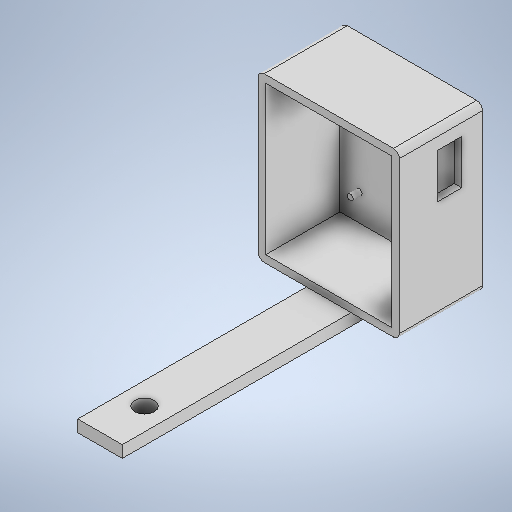
# Autodesk Inventor part: a4988_box
Saved by Autodesk Inventor 2025 (Build 290162000, 162)
## iProperties
Created: 2025-03-03
Part Number: a4988_box
Material: Všeobecné
Document SubType Name: Modeling
Designer: lukas
Density: 1 g/cm^3
Appearance: Výchozí
Author: lukas
## iProperties of the stored document a4988_box_3D tisk.ipt
Created: 2025-03-03
Part Number: a4988_box_3D tisk
Material: Všeobecné
Document SubType Name: Modeling
Designer: lukas
Density: 1 g/cm^3
Appearance: Výchozí
Author: lukas
Autodesk Inventor part; units mm, degrees
ref_plane "YZ Plane" through (0, 0, 0) normal (1, 0, 0) x (0, 1, 0)
ref_plane "XZ Plane" through (0, 0, 0) normal (0, 1, 0) x (-1, 0, 0)
ref_plane "XY Plane" through (0, 0, 0) normal (0, 0, 1) x (1, 0, 0)
sketch "Náčrt1" plane through (0, 0, 0) normal (0, 0, 1) x (1, 0, 0)
  line L0 (-21.25, 25) -> (21.25, 25)
  line L1 (21.25, 25) -> (21.25, -25)
  line L2 (21.25, -25) -> (-21.25, -25)
  line L3 (-21.25, -25) -> (-21.25, 25)
  line L4 (0, 35) -> (0, -35) projected
  line L5 (-29.75, 0) -> (29.75, 0) projected
  point P0 (0, 0)
  dimension "d0" = 50
  dimension "d1" = 42.5
  constraints: 8 end point, 2 parallel, 1 horizontal, 1 perpendicular, 2 other
  measures "d0" distance between parallel lines of L2 L0
  measures "d1" distance between parallel lines of L3 L1
extrude "Vysunutí1" add sketch "Náčrt1" along normal blind 3
sketch "Náčrt2" plane through (0, 0, 3) normal (0, 0, 1) x (1, 0, 0)
  line L0 (0, 35) -> (0, -35) projected
  line L1 (-29.75, 0) -> (29.75, 0) projected
  line L2 (21.25, -25) -> (21.25, 25) projected
  line L3 (21.25, 25) -> (-21.25, 25) projected
  line L4 (-21.25, 25) -> (-21.25, -25) projected
  line L5 (-21.25, -25) -> (21.25, -25) projected
  line L6 (-17.5, 21.5) -> (17.5, 21.5) construction
  line L7 (17.5, 21.5) -> (17.5, -21.5) construction
  line L8 (17.5, -21.5) -> (-17.5, -21.5) construction
  line L9 (-17.5, -21.5) -> (-17.5, 21.5) construction
  circle A0 centre (-14.75, 16) radius 1
  circle A1 centre (-14.75, -16) radius 1
  point P0 (0, 0)
  dimension "d4" = 35
  dimension "d5" = 43
  dimension "d6" = 2
  dimension "d9" = 16
  dimension "d10" = 36
  constraints: 8 end point, 2 centre point, 2 parallel, 1 horizontal, 1 perpendicular, 1 symmetric about line, 3 other
  measures "d4" distance of L6.start L6.end
  measures "d5" distance of L6.end L7.end
  measures "d6" diameter of A0
  measures "d9" distance from line of L1 A0.centre
  measures "d10" distance from line of L2 A0.centre
extrude "Vysunutí2" add sketch "Náčrt2" along normal blind 3 contours A0 | A1
sketch "Náčrt3" plane through (0, 0, 3) normal (0, 0, 1) x (1, 0, 0)
  circle A0 centre (-14.75, -16) radius 1 projected
  circle A1 centre (-14.75, 16) radius 1 projected
  line L0 (21.25, -25) -> (21.25, 25) projected
  line L1 (21.25, 25) -> (-21.25, 25) projected
  line L2 (-21.25, 25) -> (-21.25, -25) projected
  line L3 (-21.25, -25) -> (21.25, -25) projected
  line L4 (0, 35) -> (0, -35) projected
  line L5 (-29.75, 0) -> (29.75, 0) projected
  line L6 (-23.75, 27.5) -> (23.75, 27.5)
  line L7 (23.75, 27.5) -> (23.75, -27.5)
  line L8 (23.75, -27.5) -> (-23.75, -27.5)
  line L9 (-23.75, -27.5) -> (-23.75, 27.5)
  line L10 (-21.25, 25) -> (21.25, 25)
  line L11 (21.25, 25) -> (21.25, -25)
  line L12 (21.25, -25) -> (-21.25, -25)
  line L13 (-21.25, -25) -> (-21.25, 25)
  point P0 (0, 0)
  dimension "d13" = 2.5
  constraints: 16 end point, 2 parallel, 1 horizontal, 1 perpendicular, 3 other
  measures "d13" distance between parallel lines of L1 L6
extrude "Vysunutí3" add sketch "Náčrt3" along normal blind 25 and the other way blind 3 contours L0 L5 L7 L8 L4 L3 | L0 L1 L4 L6 L7 L5 | L4 L8 L9 L5 L2 L3 | L1 L2 L5 L9 L6 L4
sketch "Náčrt4" plane through (23.75, -27.5, 28) normal (1, 0, 0) x (0, 0, -1)
  line L0 (13, 34) -> (21, 34)
  line L1 (21, 34) -> (21, 49)
  line L2 (21, 49) -> (13, 49)
  line L3 (13, 49) -> (13, 34)
  line L4 (0, 55) -> (28, 55) projected
  line L5 (0, 0) -> (0, 55) projected
  line L6 (28, 0) -> (0, 0) projected
  line L7 (28, 55) -> (28, 0) projected
  line L8 (-6.6, 27.5) -> (39.6, 27.5) projected
  line L9 (28, -11) -> (28, 66) projected
  line L10 (25, 2.5) -> (25, 52.5) projected
  line L11 (0, 52.5) -> (25, 52.5) projected
  point P0 (28, 27.5)
  dimension "d18" = 15
  dimension "d19" = 8
  dimension "d20" = 7
  dimension "d21" = 6
  constraints: 8 end point, 2 parallel, 1 horizontal, 1 perpendicular
  measures "d18" distance of L2.end L0.start
  measures "d19" distance of L0.start L0.end
  measures "d20" distance between parallel lines of L7 L1
  measures "d21" distance between parallel lines of L4 L2
extrude "Vysunutí4" cut sketch "Náčrt4" against normal up to surface (2.5 mm away) contours L3 L2 L1 L0
sketch "Náčrt5" plane through (-23.75, -27.5, 28) normal (0, -1, 0) x (1, 0, 0)
  line L0 (47.5, -28) -> (47.5, 0) projected
  line L1 (0, 0) -> (47.5, 0) projected
  line L2 (0, -28) -> (0, 0) projected
  line L3 (47.5, -28) -> (0, -28) projected
  line L4 (23.75, 99) -> (23.75, -55) projected
  line L5 (-9.5, -28) -> (57, -28) projected
  line L6 (31.25, -28) -> (16.25, -28)
  line L7 (16.25, -28) -> (16.25, 77)
  line L8 (16.25, 77) -> (31.25, 77)
  line L9 (31.25, 77) -> (31.25, -28)
  point P0 (23.75, -28)
  point P1 (31.25, -28)
  dimension "d24" = 15
  dimension "d25" = 77
  constraints: 8 end point, 2 parallel, 1 horizontal, 1 perpendicular, 1 point on line, 1 other
  measures "d24" distance between parallel lines of L9 L7
  measures "d25" distance between parallel lines of L1 L8
extrude "Vysunutí5" add sketch "Náčrt5" along normal blind 5 contours L3 L4 L1 L9 | L1 L4 L8 L9 | L3 L7 L1 L4 | L1 L7 L8 L4
sketch "Náčrt6" plane through (-23.75, -32.5, 28) normal (0, -1, 0) x (1, 0, 0)
  line L0 (16.25, 77) -> (16.25, -28) projected
  line L1 (16.25, -28) -> (31.25, -28) projected
  line L2 (31.25, -28) -> (31.25, 77) projected
  line L3 (31.25, 77) -> (16.25, 77) projected
  line L4 (23.75, 99) -> (23.75, -55) projected
  line L5 (-9.5, -28) -> (57, -28) projected
  point P0 (23.75, -28)
  point P1 (23.75, 62)
  dimension "d28" = 15
  constraints: 1 point on line
  measures "d28" distance from line of L3 point (23.75, 62)
hole "Díra1" at (0, -32.5, 90) direction (0, 1, 0) diameter 6.6 end through all
chamfer "Zkosení1" distance 1 angle 45 4 edges at (-7.5, -32.5, 52.5) (7.5, -32.5, 52.5) (0, -32.5, 105) (0, -32.5, 0)
fillet "Zaoblení1" radius 2 4 edges at (-23.75, -27.5, 14) (23.75, -27.5, 14) (23.75, 27.5, 14) (-23.75, 27.5, 14)
